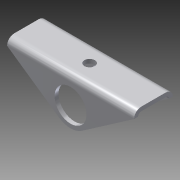
# Autodesk Inventor part: Pipe to Gas Spring Connector (9417K91)
Saved by Autodesk Inventor 2014 (Build 180170000, 170)
## iProperties
Created: 2014-01-12
Part Number: Pipe to Gas Spring Connector (9417K91)
Material: Aluminum
Document SubType Name: Sheet Metal
Designer: Michael
Density: 2.71 g/cm^3
Sheet Metal Rule: Default
Appearance: Satin
Author: Michael
Autodesk Inventor part; units mm, degrees
ref_plane "YZ Plane" through (0, 0, 0) normal (1, 0, 0) x (0, 1, 0)
ref_plane "XZ Plane" through (0, 0, 0) normal (0, 1, 0) x (-1, 0, 0)
ref_plane "XY Plane" through (0, 0, 0) normal (0, 0, 1) x (1, 0, 0)
sketch "Sketch1" plane through (0, 0, 0) normal (0, 0, 1) x (1, 0, 0)
  arc A0 (0, 6.3881) -> (0, -6.3881) centre (0, 0) ccw
  line L0 (-25.4, 7.9375) -> (-4.5511, -6.5496)
  line L1 (0, 7.9375) -> (0, -13.1033) construction
  line L2 (-25.4, 7.9375) -> (0, 7.9375)
  arc A1 (-4.5511, -6.5496) -> (0, -7.9756) centre (0, 0) ccw
  arc A2 (0, -6.3881) -> (0, 6.3881) centre (0, 0) ccw
  line L3 (25.4, 7.9375) -> (4.5511, -6.5496)
  line L4 (25.4, 7.9375) -> (0, 7.9375)
  arc A3 (0, -7.9756) -> (4.5511, -6.5496) centre (0, 0) ccw
  dimension "d0" = 12.7762
  dimension "d1" = 7.9375
  dimension "d2" = 25.4
  dimension "d3" = 1.5875
  measures "d0" diameter of A0
  measures "d1" distance from line of point (0, 0) L2
  measures "d2" horizontal distance of point (0, 0) L0.start
  measures "d3" radial gap between concentric circles of A0 A1
extrude "Plate1" add sketch "Sketch1" along normal blind 1.5875
sketch "Sketch2" plane through (25.4, 9.2075, -1.27) normal (0, 1, 0) x (-1, 0, 0)
  line L0 (50.8, 0) -> (0, 0)
  line L1 (0, 0) -> (0, -9.8425)
  line L2 (0, -9.8425) -> (50.8, -9.8425)
  line L3 (50.8, -9.8425) -> (50.8, 0)
  constraints: 6 end point, 1 horizontal, 1 perpendicular, 1 vertical
edge flange "Flange1" height 12.7 angle 90 thickness 1.5875 bend radius 1.27 thickness toward (0, 1, 0) relief tear relief width 1.5875 relief depth 0.7937 edges at (-12.7, 7.9375, 0) wall of the first edge with corners at (-25.4, 9.2075, -1.27) (25.4, 9.2075, -1.27) (25.4, 9.2075, -11.1125) (-25.4, 9.2075, -11.1125)
bend "Bend1"
corner "Corner1"
sketch "Sketch3" plane through (-25.4, 10.795, -11.1125) normal (0, 1, 0) x (1, 0, 0)
  line L0 (0, -9.8425) -> (50.8, -9.8425) projected
  line L1 (50.8, 0) -> (50.8, -9.8425) projected
  line L2 (25.4, -6.2418) -> (25.4, -0.3175) construction
  circle A0 centre (25.4, -5.08) radius 2.0828
  dimension "d35" = 4.1656
  dimension "d36" = 4.7625
  dimension "d37" = 25.4
  constraints: 2 end point, 1 centre point, 1 vertical
  measures "d35" diameter of A0
  measures "d36" distance from line of L0 A0.centre
  measures "d37" distance from line of L1 A0.centre
extrude "Cut1" cut sketch "Sketch3" against normal blind 1.5875
sketch "Sketch4" plane through (25.4, 7.9375, -12.3825) normal (0, 0, -1) x (-1, 0, 0)
  line L0 (50.8, 0) -> (0, 0)
  line L1 (0, 0) -> (0, -16.2306)
  line L2 (0, -16.2306) -> (50.8, -16.2306)
  line L3 (50.8, -16.2306) -> (50.8, 0)
  constraints: 6 end point, 1 horizontal, 1 perpendicular, 1 vertical
edge flange "Flange2" height 19.0881 angle 90 thickness 1.5875 bend radius 1.27 thickness toward (0, 0, -1) relief tear relief width 1.5875 relief depth 0.7937 edges at (0, 9.2075, -11.1125) wall of the first edge with corners at (-25.4, 7.9375, -12.3825) (25.4, 7.9375, -12.3825) (25.4, -8.2931, -12.3825) (-25.4, -8.2931, -12.3825)
bend "Bend2"
corner "Corner2"
sketch "Sketch5" plane through (25.4, -8.2931, -13.97) normal (0, 0, -1) x (-1, 0, 0)
  line L0 (50.8, 16.2306) -> (0, 16.2306) projected
  line L1 (0, 0) -> (0, 16.2306) projected
  line L2 (50.8, 0) -> (0, 0) projected
  line L3 (50.8, 16.2306) -> (50.8, 0) projected
  circle A0 centre (25.4, 8.2931) radius 6.3881 projected
  line L4 (50.8, 16.2306) -> (29.9511, 1.7435) projected
  line L5 (0, 16.2306) -> (50.8, 16.2306) projected
  line L6 (20.8489, 1.7435) -> (0, 16.2306) projected
  arc A1 (20.8489, 1.7435) -> (29.9511, 1.7435) centre (25.4, 8.2931) ccw projected
extrude "Cut2" cut sketch "Sketch5" against normal blind 1.5875 contours L3 L2 L1 L6 A1 L4 | A0
equation "\"d37\" = d2"
equation "\"d18\" = Thickness"
equation "\"d49\" = Thickness"
equation "\"d5\" = BendReliefWidth"
equation "\"d6\" = BendReliefDepth"
equation "\"d7\" = MinimumRemnant"
equation "\"d8\" = BendRadius"
equation "\"d12\" = CornerReliefSize"
equation "\"d13\" = GapSize"
equation "\"d14\" = JacobiRadiusSize"
equation "\"d39\" = BendReliefWidth"
equation "\"d40\" = BendReliefDepth"
equation "\"d41\" = MinimumRemnant"
equation "\"d42\" = BendRadius"
equation "\"d46\" = CornerReliefSize"
equation "\"d47\" = GapSize"
equation "\"d48\" = JacobiRadiusSize"
equation "\"BendRadius\" = Thickness"
equation "\"BendReliefWidth\" = Thickness"
equation "\"BendReliefDepth\" = 0.5 * Thickness"
equation "\"CornerReliefSize\" = 4 * Thickness"
equation "\"MinimumRemnant\" = 2 * Thickness"
equation "\"TransitionRadius\" = BendRadius"
equation "\"JacobiRadiusSize\" = BendRadius"
equation "\"GapSize\" = Thickness"
equation "\"d4\" = BendRadius"
equation "\"Thickness\" = 1.5875"
body "Solid1"
